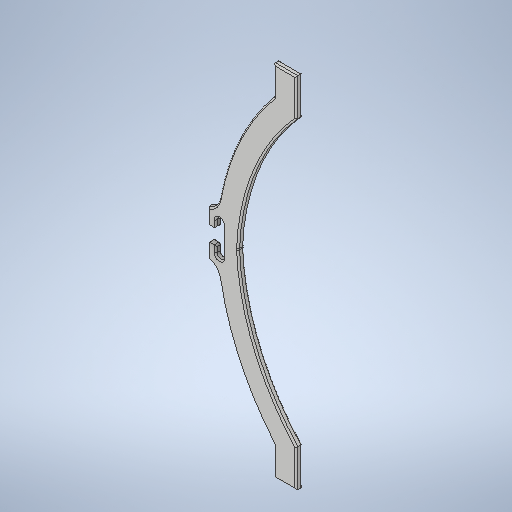
# Autodesk Inventor part: Baseplate_aussen_unten
Saved by Autodesk Inventor 2025 (Build 290162000, 162)
## iProperties
Created: 2020-01-15
Part Number: Baseplate_aussen_unten
Material: Generisch
Document SubType Name: Modeling
Designer: maxse
Density: 1 g/cm^3
Appearance: Vorgabe
Author: maxse
Autodesk Inventor part; units mm, degrees
ref_plane "YZ Plane" through (0, 0, 0) normal (1, 0, 0) x (0, 1, 0)
ref_plane "XZ Plane" through (0, 0, 0) normal (0, 1, 0) x (-1, 0, 0)
ref_plane "XY Plane" through (0, 0, 0) normal (0, 0, 1) x (1, 0, 0)
sketch "Skizze1" plane through (0, 0, 0) normal (0, 1, 0) x (-1, 0, 0)
  arc A0 (39, 0) -> (0, 95) centre (-110.879, -6.024) ccw
  line L0 (0, 95) -> (0, 120)
  line L1 (0, 120) -> (15, 120)
  line L2 (15, 120) -> (15, 100.6336)
  arc A1 (54, 0) -> (15, 100.6336) centre (-110.879, -6.024) ccw
  line L3 (39, 0) -> (54, 0)
  line L4 (0, 0) -> (39, 0)
  line L5 (59, 0) -> (59, 15)
  line L6 (59, 15) -> (52.765, 15)
  line L7 (59, 0) -> (54, 0)
  dimension "d0" = 25
  dimension "d2" = 15
  dimension "d4" = 54
  dimension "d5" = 0
  dimension "d6" = 120
  dimension "d7" = 150
  dimension "d9" = 5
  dimension "d10" = 15
  dimension "d11" = 15
  constraints: 16 end point, 6 point on circle, 3 perpendicular, 2 centre point, 2 horizontal, 2 vertical, 1 collinear, 1 concentric
  measures "d0" distance of L0.start L0.end
  measures "d2" distance of L0.end L1.end
  measures "d4" distance of L3.end L4.start
  measures "d5" distance from line of L4.start L0
  measures "d6" distance from line of L4.start L1
  measures "d7" radius of A0
  measures "d9" distance of L3.end L5.start
  measures "d10" distance of L3.end L3.start
  measures "d11" distance of L5.start L5.end
extrude "Extrusion1" add sketch "Skizze1" along normal blind 4
mirror "Spiegeln1" about plane through (-54, 0, 0) normal (0, 0, -1) of "Extrusion1"
sketch "Skizze2" plane through (0, 0, 0) normal (0, -1, 0) x (1, 0, 0)
  line L0 (-59, 15) -> (-59, -15) projected
  line L1 (-59, -5) -> (-54, -5)
  line L2 (-54, -5) -> (-54, -9.5)
  line L3 (-59, 5) -> (-54, 5)
  line L4 (-54, 5) -> (-54, 9.5)
  line L5 (-49, -9.5) -> (-49, 9.5)
  arc A0 (-49, 9.5) -> (-54, 9.5) centre (-51.5, 9.5) ccw
  arc A1 (-54, -9.5) -> (-49, -9.5) centre (-51.5, -9.5) ccw
  point P0 (0, 0)
  dimension "d15" = 10
  dimension "d16" = 5
  dimension "d17" = 10
  dimension "d18" = 5
  dimension "d19" = 5
  dimension "d20" = 24
  dimension "d21" = 4.5
  constraints: 10 end point, 4 point on circle, 4 tangent, 2 centre point, 2 horizontal, 2 point on line, 2 vertical, 1 perpendicular
  measures "d15" distance between parallel lines of L5 L0
  measures "d16" distance between parallel lines of L5 L2
  measures "d17" distance between parallel lines of L3 L1
  measures "d18" distance of L3.start L3.end
  measures "d19" distance from line of point (0, 0) L3
  measures "d21" distance from line of L1 A1.centre
extrude "Extrusion2" cut sketch "Skizze2" against normal blind 4
fillet "Rundung1" radius 10 3 edges at (-52.765, 2, -15) (-52.765, 2, 15) (-39, 2, 0)
fillet "Rundung2" radius 1 46 edges at (-7.5, 4, -120) (0, 4, -107.5) (-15, 4, -110.3168) (-7.5, 0, -120) (0, 0, -107.5) (-15, 0, -110.3168) (-54.0935, 4, -17.8718) (-38.4134, 4, -64.2123) (-54.0935, 0, -17.8718) (-38.4134, 0, -64.2123) (-38.9913, 4, 0) (-27.8012, 4, 51.1406) (-27.8012, 4, -51.1406) (-38.9913, 0, 0) (-27.8012, 0, 51.1406) (-27.8012, 0, -51.1406) (-54.0935, 4, 17.8718) (-38.4134, 4, 64.2123) (-54.0935, 0, 17.8718) (-38.4134, 0, 64.2123) (-59, 4, 10) (-59, 0, 10) (-59, 0, -10) (-59, 4, -10) (-59, 2, -5) (-59, 2, 5) (-54, 2, 5) (-54, 2, -5) (-56.5, 4, -5) (-56.5, 4, 5) (-51.5, 4, 12) (-54, 4, 7.25) (-51.5, 4, -12) (-54, 4, -7.25) (-49, 4, 0) (-51.5, 0, -12) (-54, 0, -7.25) (-51.5, 0, 12) (-54, 0, 7.25) (-49, 0, 0) (-15, 4, 110.3168) (-15, 0, 110.3168) (-7.5, 4, 120) (-7.5, 0, 120) (0, 0, 107.5) (0, 4, 107.5)
sketch "Skizze3" plane through (0, 4, 0) normal (0, 1, 0) x (1, 0, 0)
  arc A0 (0, 94.8126) -> (0, -95) centre (94.4443, -0.0937) ccw
  spline S0 degree 2 poles (-37.712, -45.9787) (-37.4072, -45.8685) (-36.7799, -45.8874) (-36.5192, -46.0129) knots 0 0 0 1 2 2 2
  spline S1 degree 2 poles (-36.5192, -46.0129) (-36.191, -46.17) (-35.705, -46.7397) (-35.5232, -47.2427) knots 0 0 0 1 2 2 2
  line L0 (-35.5232, -47.2427) -> (-35.3317, -47.7723)
  line L1 (-35.3317, -47.7723) -> (-33.5789, -47.1388)
  line L2 (-33.5789, -47.1388) -> (-33.353, -47.7637)
  line L3 (-33.353, -47.7637) -> (-38.0552, -49.4633)
  line L4 (-38.0552, -49.4633) -> (-38.4822, -48.282)
  spline S2 degree 2 poles (-38.4822, -48.282) (-38.6337, -47.8629) (-38.7087, -47.2265) (-38.6337, -46.9452) knots 0 0 0 1 2 2 2
  spline S3 degree 2 poles (-38.6337, -46.9452) (-38.5496, -46.6175) (-38.1045, -46.1206) (-37.712, -45.9787) knots 0 0 0 1 2 2 2
  spline S4 degree 2 poles (-37.4574, -46.6234) (-37.7013, -46.7116) (-37.9989, -47.0087) (-38.0513, -47.2215) knots 0 0 0 1 2 2 2
  spline S5 degree 2 poles (-38.0513, -47.2215) (-38.0966, -47.4059) (-38.0334, -47.8311) (-37.9273, -48.1246) knots 0 0 0 1 2 2 2
  line L5 (-37.9273, -48.1246) -> (-37.74, -48.6428)
  line L6 (-37.74, -48.6428) -> (-35.8652, -47.9652)
  line L7 (-35.8652, -47.9652) -> (-36.0195, -47.5384)
  spline S6 degree 2 poles (-36.0195, -47.5384) (-36.1572, -47.1573) (-36.4486, -46.7327) (-36.6637, -46.6381) knots 0 0 0 1 2 2 2
  spline S7 degree 2 poles (-36.6637, -46.6381) (-36.8557, -46.5481) (-37.2326, -46.5422) (-37.4574, -46.6234) knots 0 0 0 1 2 2 2
  spline S8 degree 2 poles (-35.6468, -42.3782) (-35.5687, -42.4335) (-35.2949, -42.616) (-35.199, -42.7123) knots 0 0 0 1 2 2 2
  spline S9 degree 2 poles (-35.199, -42.7123) (-35.0622, -42.842) (-34.8756, -43.1089) (-34.7865, -43.3781) knots 0 0 0 1 2 2 2
  spline S10 degree 2 poles (-34.7865, -43.3781) (-34.7139, -43.5974) (-34.7482, -44.0483) (-34.8485, -44.248) knots 0 0 0 1 2 2 2
  spline S11 degree 2 poles (-34.8485, -44.248) (-34.9476, -44.4387) (-35.3211, -44.7544) (-35.5596, -44.8334) knots 0 0 0 1 2 2 2
  spline S12 degree 2 poles (-35.5596, -44.8334) (-35.9288, -44.9556) (-36.5551, -44.8173) (-36.8172, -44.5284) knots 0 0 0 1 2 2 2
  spline S13 degree 2 poles (-36.8172, -44.5284) (-37.055, -44.2742) (-37.4288, -43.4932) (-37.6124, -43.0289) knots 0 0 0 1 2 2 2
  line L8 (-37.6124, -43.0289) -> (-37.7278, -43.0671)
  spline S14 degree 2 poles (-37.7278, -43.0671) (-37.9355, -43.1359) (-38.1512, -43.3482) (-38.1861, -43.4878) knots 0 0 0 1 2 2 2
  spline S15 degree 2 poles (-38.1861, -43.4878) (-38.2209, -43.6274) (-38.1576, -43.9734) (-38.099, -44.1504) knots 0 0 0 1 2 2 2
  spline S16 degree 2 poles (-38.099, -44.1504) (-38.0302, -44.3581) (-37.7212, -44.8789) (-37.509, -45.1203) knots 0 0 0 1 2 2 2
  line L9 (-37.509, -45.1203) -> (-37.4976, -45.1549)
  line L10 (-37.4976, -45.1549) -> (-38.1092, -45.3574)
  spline S17 degree 2 poles (-38.1092, -45.3574) (-38.2101, -45.2072) (-38.5305, -44.6261) (-38.6311, -44.3223) knots 0 0 0 1 2 2 2
  spline S18 degree 2 poles (-38.6311, -44.3223) (-38.7534, -43.953) (-38.8048, -43.4109) (-38.721, -43.1612) knots 0 0 0 1 2 2 2
  spline S19 degree 2 poles (-38.721, -43.1612) (-38.6398, -42.9166) (-38.238, -42.5702) (-37.9033, -42.4594) knots 0 0 0 1 2 2 2
  line L11 (-37.9033, -42.4594) -> (-35.4685, -41.6534)
  line L12 (-35.4685, -41.6534) -> (-35.2698, -42.2534)
  line L13 (-35.2698, -42.2534) -> (-35.6468, -42.3782)
  line L14 (-36.1468, -42.5438) -> (-37.1354, -42.871)
  spline S20 degree 2 poles (-37.1354, -42.871) (-37.0449, -43.0801) (-36.7642, -43.7085) (-36.6352, -43.892) knots 0 0 0 1 2 2 2
  spline S21 degree 2 poles (-36.6352, -43.892) (-36.4832, -44.1063) (-36.0761, -44.3172) (-35.8069, -44.2281) knots 0 0 0 1 2 2 2
  spline S22 degree 2 poles (-35.8069, -44.2281) (-35.4992, -44.1262) (-35.3022, -43.6769) (-35.4117, -43.3461) knots 0 0 0 1 2 2 2
  spline S23 degree 2 poles (-35.4117, -43.3461) (-35.5047, -43.0653) (-35.8998, -42.6839) (-36.1468, -42.5438) knots 0 0 0 1 2 2 2
  line L15 (-39.2549, -39.8049) -> (-39.2454, -39.8359)
  spline S24 degree 2 poles (-39.2454, -39.8359) (-39.2434, -39.9116) (-39.2049, -40.0651) (-39.1728, -40.1697) knots 0 0 0 1 2 2 2
  spline S25 degree 2 poles (-39.1728, -40.1697) (-39.098, -40.4137) (-38.7377, -40.8288) (-38.462, -40.9816) knots 0 0 0 1 2 2 2
  line L16 (-38.462, -40.9816) -> (-35.9168, -40.2016)
  line L17 (-35.9168, -40.2016) -> (-35.7316, -40.806)
  line L18 (-35.7316, -40.806) -> (-39.3189, -41.9054)
  line L19 (-39.3189, -41.9054) -> (-39.5042, -41.301)
  line L20 (-39.5042, -41.301) -> (-38.9695, -41.1372)
  spline S26 degree 2 poles (-38.9695, -41.1372) (-39.3649, -40.8981) (-39.7559, -40.4797) (-39.8271, -40.2473) knots 0 0 0 1 2 2 2
  spline S27 degree 2 poles (-39.8271, -40.2473) (-39.8556, -40.1543) (-39.8763, -40.0589) (-39.8825, -39.9973) knots 0 0 0 1 2 2 2
  line L21 (-39.8825, -39.9973) -> (-39.2549, -39.8049)
  line L22 (-36.6281, -37.8134) -> (-36.4518, -38.4205)
  line L23 (-36.4518, -38.4205) -> (-40.0551, -39.4665)
  line L24 (-40.0551, -39.4665) -> (-40.2313, -38.8594)
  line L25 (-40.2313, -38.8594) -> (-36.6281, -37.8134)
  line L26 (-40.843, -38.9906) -> (-40.6431, -39.6793)
  line L27 (-40.6431, -39.6793) -> (-41.2734, -39.8623)
  line L28 (-41.2734, -39.8623) -> (-41.4734, -39.1736)
  line L29 (-41.4734, -39.1736) -> (-40.843, -38.9906)
  spline S28 degree 2 poles (-37.0651, -35.9211) (-36.9663, -36.2847) (-36.9906, -36.9674) (-37.0437, -37.2044) knots 0 0 0 1 2 2 2
  line L30 (-37.0437, -37.2044) -> (-37.7279, -37.3905)
  line L31 (-37.7279, -37.3905) -> (-37.7364, -37.3592)
  spline S29 degree 2 poles (-37.7364, -37.3592) (-37.6951, -37.264) (-37.604, -37.0124) (-37.5697, -36.8142) knots 0 0 0 1 2 2 2
  spline S30 degree 2 poles (-37.5697, -36.8142) (-37.5369, -36.6415) (-37.5295, -36.2364) (-37.5837, -36.037) knots 0 0 0 1 2 2 2
  spline S31 degree 2 poles (-37.5837, -36.037) (-37.6231, -35.8923) (-37.7799, -35.578) (-37.8559, -35.5147) knots 0 0 0 1 2 2 2
  spline S32 degree 2 poles (-37.8559, -35.5147) (-37.961, -35.4215) (-38.1568, -35.3656) (-38.3288, -35.4124) knots 0 0 0 1 2 2 2
  spline S33 degree 2 poles (-38.3288, -35.4124) (-38.5439, -35.4709) (-38.7029, -35.766) (-38.6954, -36.0873) knots 0 0 0 1 2 2 2
  spline S34 degree 2 poles (-38.6954, -36.0873) (-38.6908, -36.212) (-38.667, -36.6087) (-38.6664, -36.7807) knots 0 0 0 1 2 2 2
  spline S35 degree 2 poles (-38.6664, -36.7807) (-38.6749, -37.2281) (-39.0733, -37.7395) (-39.4291, -37.8363) knots 0 0 0 1 2 2 2
  spline S36 degree 2 poles (-39.4291, -37.8363) (-39.9217, -37.9702) (-40.7365, -37.3982) (-40.9024, -36.7883) knots 0 0 0 1 2 2 2
  spline S37 degree 2 poles (-40.9024, -36.7883) (-40.9842, -36.4872) (-41.0015, -35.8369) (-40.9445, -35.5988) knots 0 0 0 1 2 2 2
  line L32 (-40.9445, -35.5988) -> (-40.2916, -35.4212)
  line L33 (-40.2916, -35.4212) -> (-40.283, -35.4525)
  spline S38 degree 2 poles (-40.283, -35.4525) (-40.4069, -35.7381) (-40.4667, -36.3675) (-40.387, -36.6607) knots 0 0 0 1 2 2 2
  spline S39 degree 2 poles (-40.387, -36.6607) (-40.3051, -36.9618) (-39.9383, -37.3071) (-39.6841, -37.238) knots 0 0 0 1 2 2 2
  spline S40 degree 2 poles (-39.6841, -37.238) (-39.4535, -37.1753) (-39.2976, -36.8683) (-39.3016, -36.5755) knots 0 0 0 1 2 2 2
  spline S41 degree 2 poles (-39.3016, -36.5755) (-39.3026, -36.433) (-39.3236, -36.0776) (-39.3306, -35.8821) knots 0 0 0 1 2 2 2
  spline S42 degree 2 poles (-39.3306, -35.8821) (-39.3374, -35.4557) (-38.9827, -34.9225) (-38.58, -34.813) knots 0 0 0 1 2 2 2
  spline S43 degree 2 poles (-38.58, -34.813) (-38.3454, -34.7492) (-37.881, -34.8203) (-37.6796, -34.9587) knots 0 0 0 1 2 2 2
  spline S44 degree 2 poles (-37.6796, -34.9587) (-37.4672, -35.1067) (-37.1661, -35.5497) (-37.0651, -35.9211) knots 0 0 0 1 2 2 2
  line L34 (-38.8586, -29.0048) -> (-38.2094, -31.8282)
  line L35 (-38.2094, -31.8282) -> (-43.0823, -32.9486)
  line L36 (-43.0823, -32.9486) -> (-43.2312, -32.301)
  line L37 (-43.2312, -32.301) -> (-38.9349, -31.3132)
  line L38 (-38.9349, -31.3132) -> (-39.4351, -29.1374)
  line L39 (-39.4351, -29.1374) -> (-38.8586, -29.0048)
  spline S45 degree 2 poles (-41.4057, -25.8908) (-40.4764, -25.7027) (-39.2828, -26.3912) (-39.1316, -27.1378) knots 0 0 0 1 2 2 2
  spline S46 degree 2 poles (-39.1316, -27.1378) (-38.9765, -27.9042) (-39.8432, -28.9934) (-40.7407, -29.1751) knots 0 0 0 1 2 2 2
  spline S47 degree 2 poles (-40.7407, -29.1751) (-41.662, -29.3616) (-42.866, -28.6628) (-43.0156, -27.9242) knots 0 0 0 1 2 2 2
  spline S48 degree 2 poles (-43.0156, -27.9242) (-43.1667, -27.1776) (-42.331, -26.0782) (-41.4057, -25.8908) knots 0 0 0 1 2 2 2
  spline S49 degree 2 poles (-41.2762, -26.5302) (-41.9911, -26.675) (-42.5807, -27.3359) (-42.4834, -27.8164) knots 0 0 0 1 2 2 2
  spline S50 degree 2 poles (-42.4834, -27.8164) (-42.3861, -28.297) (-41.585, -28.6805) (-40.8702, -28.5357) knots 0 0 0 1 2 2 2
  spline S51 degree 2 poles (-40.8702, -28.5357) (-40.1752, -28.395) (-39.5665, -27.7261) (-39.6638, -27.2455) knots 0 0 0 1 2 2 2
  spline S52 degree 2 poles (-39.6638, -27.2455) (-39.7603, -26.769) (-40.5693, -26.3871) (-41.2762, -26.5302) knots 0 0 0 1 2 2 2
  line L40 (-40.1779, -22.0386) -> (-40.0696, -22.6614)
  line L41 (-40.0696, -22.6614) -> (-40.4449, -22.7266)
  spline S53 degree 2 poles (-40.4449, -22.7266) (-40.3001, -22.8495) (-40.1037, -23.0333) (-40.0108, -23.1652) knots 0 0 0 1 2 2 2
  spline S54 degree 2 poles (-40.0108, -23.1652) (-39.924, -23.2859) (-39.8069, -23.5575) (-39.7743, -23.7451) knots 0 0 0 1 2 2 2
  spline S55 degree 2 poles (-39.7743, -23.7451) (-39.7215, -24.0485) (-39.8841, -24.6032) (-40.0964, -24.8252) knots 0 0 0 1 2 2 2
  spline S56 degree 2 poles (-40.0964, -24.8252) (-40.3087, -25.0472) (-40.9925, -25.3717) (-41.4596, -25.4529) knots 0 0 0 1 2 2 2
  spline S57 degree 2 poles (-41.4596, -25.4529) (-41.9466, -25.5376) (-42.7009, -25.4097) (-43.0066, -25.2366) knots 0 0 0 1 2 2 2
  spline S58 degree 2 poles (-43.0066, -25.2366) (-43.2815, -25.0747) (-43.6562, -24.5517) (-43.711, -24.2364) knots 0 0 0 1 2 2 2
  spline S59 degree 2 poles (-43.711, -24.2364) (-43.7589, -23.9609) (-43.7067, -23.5282) (-43.6185, -23.2785) knots 0 0 0 1 2 2 2
  line L42 (-43.6185, -23.2785) -> (-45.2153, -23.5561)
  line L43 (-45.2153, -23.5561) -> (-45.3236, -22.9334)
  line L44 (-45.3236, -22.9334) -> (-40.1779, -22.0386)
  line L45 (-40.9678, -22.8176) -> (-43.1035, -23.1889)
  spline S60 degree 2 poles (-43.1035, -23.1889) (-43.175, -23.4399) (-43.195, -23.8217) (-43.1582, -24.0333) knots 0 0 0 1 2 2 2
  spline S61 degree 2 poles (-43.1582, -24.0333) (-43.0749, -24.5123) (-42.262, -24.9303) (-41.5833, -24.8123) knots 0 0 0 1 2 2 2
  spline S62 degree 2 poles (-41.5833, -24.8123) (-40.9287, -24.6985) (-40.3102, -24.1632) (-40.3901, -23.7041) knots 0 0 0 1 2 2 2
  spline S63 degree 2 poles (-40.3901, -23.7041) (-40.4324, -23.4606) (-40.742, -23.0045) (-40.9678, -22.8176) knots 0 0 0 1 2 2 2
  line L46 (-43.6537, -19.6231) -> (-43.6489, -19.6552)
  spline S64 degree 2 poles (-43.6489, -19.6552) (-43.6581, -19.7303) (-43.6426, -19.8878) (-43.6264, -19.996) knots 0 0 0 1 2 2 2
  spline S65 degree 2 poles (-43.6264, -19.996) (-43.5885, -20.2484) (-43.2934, -20.7122) (-43.0433, -20.904) knots 0 0 0 1 2 2 2
  line L47 (-43.0433, -20.904) -> (-40.4108, -20.5085)
  line L48 (-40.4108, -20.5085) -> (-40.3169, -21.1336)
  line L49 (-40.3169, -21.1336) -> (-44.0273, -21.6911)
  line L50 (-44.0273, -21.6911) -> (-44.1212, -21.066)
  line L51 (-44.1212, -21.066) -> (-43.5682, -20.9829)
  spline S66 degree 2 poles (-43.5682, -20.9829) (-43.9239, -20.6881) (-44.2488, -20.2165) (-44.285, -19.9761) knots 0 0 0 1 2 2 2
  spline S67 degree 2 poles (-44.285, -19.9761) (-44.2994, -19.88) (-44.3058, -19.7826) (-44.3028, -19.7207) knots 0 0 0 1 2 2 2
  line L52 (-44.3028, -19.7207) -> (-43.6537, -19.6231)
  spline S68 degree 2 poles (-42.9318, -15.8585) (-41.9912, -15.739) (-40.8513, -16.5131) (-40.7553, -17.2688) knots 0 0 0 1 2 2 2
  spline S69 degree 2 poles (-40.7553, -17.2688) (-40.6567, -18.0446) (-41.601, -19.0672) (-42.5094, -19.1826) knots 0 0 0 1 2 2 2
  spline S70 degree 2 poles (-42.5094, -19.1826) (-43.442, -19.3011) (-44.5914, -18.5159) (-44.6864, -17.7683) knots 0 0 0 1 2 2 2
  spline S71 degree 2 poles (-44.6864, -17.7683) (-44.7824, -17.0126) (-43.8683, -15.9775) (-42.9318, -15.8585) knots 0 0 0 1 2 2 2
  spline S72 degree 2 poles (-42.8496, -16.5056) (-43.5731, -16.5975) (-44.2096, -17.2135) (-44.1478, -17.6998) knots 0 0 0 1 2 2 2
  spline S73 degree 2 poles (-44.1478, -17.6998) (-44.086, -18.1862) (-43.3152, -18.6274) (-42.5917, -18.5355) knots 0 0 0 1 2 2 2
  spline S74 degree 2 poles (-42.5917, -18.5355) (-41.8882, -18.4461) (-41.2321, -17.8236) (-41.2939, -17.3373) knots 0 0 0 1 2 2 2
  spline S75 degree 2 poles (-41.2939, -17.3373) (-41.3552, -16.8549) (-42.1341, -16.4147) (-42.8496, -16.5056) knots 0 0 0 1 2 2 2
  line L53 (-41.4306, -12.0462) -> (-41.3684, -12.6752)
  line L54 (-41.3684, -12.6752) -> (-43.4973, -12.8859)
  spline S76 degree 2 poles (-43.4973, -12.8859) (-43.7554, -12.9114) (-44.1942, -13.0037) (-44.32, -13.0894) knots 0 0 0 1 2 2 2
  spline S77 degree 2 poles (-44.32, -13.0894) (-44.4536, -13.18) (-44.5635, -13.4678) (-44.5404, -13.7016) knots 0 0 0 1 2 2 2
  spline S78 degree 2 poles (-44.5404, -13.7016) (-44.5173, -13.9355) (-44.2182, -14.4067) (-43.993, -14.6247) knots 0 0 0 1 2 2 2
  line L55 (-43.993, -14.6247) -> (-41.2028, -14.3485)
  line L56 (-41.2028, -14.3485) -> (-41.1405, -14.9776)
  line L57 (-41.1405, -14.9776) -> (-44.8743, -15.3471)
  line L58 (-44.8743, -15.3471) -> (-44.9365, -14.718)
  line L59 (-44.9365, -14.718) -> (-44.5212, -14.6769)
  spline S79 degree 2 poles (-44.5212, -14.6769) (-44.8032, -14.4198) (-45.1232, -13.9018) (-45.1535, -13.5954) knots 0 0 0 1 2 2 2
  spline S80 degree 2 poles (-45.1535, -13.5954) (-45.2078, -13.047) (-44.5434, -12.3542) (-43.8539, -12.286) knots 0 0 0 1 2 2 2
  line L60 (-43.8539, -12.286) -> (-41.4306, -12.0462)
  spline S81 degree 2 poles (-41.6553, -7.2225) (-41.6322, -7.6636) (-41.8285, -8.3312) (-42.0471, -8.5739) knots 0 0 0 1 2 2 2
  spline S82 degree 2 poles (-42.0471, -8.5739) (-42.2923, -8.8505) (-43.0094, -9.103) (-43.5435, -9.131) knots 0 0 0 1 2 2 2
  line L61 (-43.5435, -9.131) -> (-46.6591, -9.2942)
  line L62 (-46.6591, -9.2942) -> (-46.6939, -8.6306)
  line L63 (-46.6939, -8.6306) -> (-43.5782, -8.4674)
  spline S83 degree 2 poles (-43.5782, -8.4674) (-43.2302, -8.4492) (-42.7655, -8.3356) (-42.5819, -8.2002) knots 0 0 0 1 2 2 2
  spline S84 degree 2 poles (-42.5819, -8.2002) (-42.3866, -8.0561) (-42.2044, -7.584) (-42.2218, -7.2522) knots 0 0 0 1 2 2 2
  spline S85 degree 2 poles (-42.2218, -7.2522) (-42.2381, -6.9406) (-42.4699, -6.4659) (-42.6792, -6.3429) knots 0 0 0 1 2 2 2
  spline S86 degree 2 poles (-42.6792, -6.3429) (-42.8759, -6.2275) (-43.3459, -6.1628) (-43.6818, -6.1804) knots 0 0 0 1 2 2 2
  line L64 (-43.6818, -6.1804) -> (-46.8136, -6.3444)
  line L65 (-46.8136, -6.3444) -> (-46.8484, -5.6808)
  line L66 (-46.8484, -5.6808) -> (-43.7327, -5.5177)
  spline S87 degree 2 poles (-43.7327, -5.5177) (-43.2107, -5.4903) (-42.4552, -5.6617) (-42.1863, -5.9155) knots 0 0 0 1 2 2 2
  spline S88 degree 2 poles (-42.1863, -5.9155) (-41.9391, -6.1419) (-41.6794, -6.7613) (-41.6553, -7.2225) knots 0 0 0 1 2 2 2
  line L67 (-41.9473, -1.5713) -> (-41.9336, -2.2032)
  line L68 (-41.9336, -2.2032) -> (-44.0725, -2.2497)
  spline S89 degree 2 poles (-44.0725, -2.2497) (-44.3317, -2.2554) (-44.7763, -2.3137) (-44.9083, -2.3895) knots 0 0 0 1 2 2 2
  spline S90 degree 2 poles (-44.9083, -2.3895) (-45.0485, -2.4695) (-45.1802, -2.748) (-45.1751, -2.9829) knots 0 0 0 1 2 2 2
  spline S91 degree 2 poles (-45.1751, -2.9829) (-45.17, -3.2179) (-44.908, -3.7107) (-44.7003, -3.9453) knots 0 0 0 1 2 2 2
  line L69 (-44.7003, -3.9453) -> (-41.897, -3.8844)
  line L70 (-41.897, -3.8844) -> (-41.8833, -4.5163)
  line L71 (-41.8833, -4.5163) -> (-45.6344, -4.5979)
  line L72 (-45.6344, -4.5979) -> (-45.6482, -3.9659)
  line L73 (-45.6482, -3.9659) -> (-45.2309, -3.9568)
  spline S92 degree 2 poles (-45.2309, -3.9568) (-45.4923, -3.6788) (-45.7715, -3.1378) (-45.7782, -2.8299) knots 0 0 0 1 2 2 2
  spline S93 degree 2 poles (-45.7782, -2.8299) (-45.7902, -2.279) (-45.0746, -1.6393) (-44.3819, -1.6242) knots 0 0 0 1 2 2 2
  line L74 (-44.3819, -1.6242) -> (-41.9473, -1.5713)
  line L75 (-41.9476, -0.0397) -> (-41.9463, -0.6718)
  line L76 (-41.9463, -0.6718) -> (-45.6984, -0.679)
  line L77 (-45.6984, -0.679) -> (-45.6996, -0.0469)
  line L78 (-45.6996, -0.0469) -> (-41.9476, -0.0397)
  line L79 (-46.3237, -0.0035) -> (-46.3223, -0.7207)
  line L80 (-46.3223, -0.7207) -> (-46.9787, -0.722)
  line L81 (-46.9787, -0.722) -> (-46.9801, -0.0048)
  line L82 (-46.9801, -0.0048) -> (-46.3237, -0.0035)
  line L83 (-45.6527, 3.8949) -> (-41.9243, 2.4195)
  line L84 (-41.9243, 2.4195) -> (-41.9336, 1.8524)
  line L85 (-41.9336, 1.8524) -> (-45.7081, 0.5121)
  line L86 (-45.7081, 0.5121) -> (-45.6969, 1.1968)
  line L87 (-45.6969, 1.1968) -> (-42.7915, 2.1744)
  line L88 (-42.7915, 2.1744) -> (-45.6634, 3.2386)
  line L89 (-45.6634, 3.2386) -> (-45.6527, 3.8949)
  spline S94 degree 2 poles (-41.729, 5.935) (-41.767, 5.0363) (-42.8167, 4.0911) (-43.7478, 4.1304) knots 0 0 0 1 2 2 2
  spline S95 degree 2 poles (-43.7478, 4.1304) (-44.6627, 4.169) (-45.7071, 5.1743) (-45.6745, 5.9475) knots 0 0 0 1 2 2 2
  spline S96 degree 2 poles (-45.6745, 5.9475) (-45.6598, 6.2957) (-45.4346, 6.8255) (-45.2117, 7.0148) knots 0 0 0 1 2 2 2
  spline S97 degree 2 poles (-45.2117, 7.0148) (-44.9886, 7.2082) (-44.3601, 7.3966) (-43.9108, 7.3776) knots 0 0 0 1 2 2 2
  line L90 (-43.9108, 7.3776) -> (-43.5667, 7.3631)
  line L91 (-43.5667, 7.3631) -> (-43.6763, 4.7682)
  spline S98 degree 2 poles (-43.6763, 4.7682) (-43.0245, 4.7406) (-42.3045, 5.3672) (-42.2799, 5.9502) knots 0 0 0 1 2 2 2
  spline S99 degree 2 poles (-42.2799, 5.9502) (-42.2712, 6.1566) (-42.3474, 6.5613) (-42.4134, 6.7263) knots 0 0 0 1 2 2 2
  spline S100 degree 2 poles (-42.4134, 6.7263) (-42.4872, 6.8998) (-42.619, 7.1406) (-42.6805, 7.2202) knots 0 0 0 1 2 2 2
  line L92 (-42.6805, 7.2202) -> (-42.679, 7.2566)
  line L93 (-42.679, 7.2566) -> (-41.9908, 7.2276)
  spline S101 degree 2 poles (-41.9908, 7.2276) (-41.9508, 7.1164) (-41.8353, 6.779) (-41.8043, 6.6479) knots 0 0 0 1 2 2 2
  spline S102 degree 2 poles (-41.8043, 6.6479) (-41.7594, 6.4635) (-41.7194, 6.1617) (-41.729, 5.935) knots 0 0 0 1 2 2 2
  spline S103 degree 2 poles (-44.0744, 6.7681) (-44.3298, 6.7708) (-44.7067, 6.6812) (-44.8364, 6.5853) knots 0 0 0 1 2 2 2
  spline S104 degree 2 poles (-44.8364, 6.5853) (-44.9827, 6.482) (-45.1471, 6.1442) (-45.1578, 5.8892) knots 0 0 0 1 2 2 2
  spline S105 degree 2 poles (-45.1578, 5.8892) (-45.1684, 5.6382) (-45.0335, 5.2797) (-44.8939, 5.1278) knots 0 0 0 1 2 2 2
  spline S106 degree 2 poles (-44.8939, 5.1278) (-44.7501, 4.9798) (-44.396, 4.8188) (-44.158, 4.7885) knots 0 0 0 1 2 2 2
  line L94 (-44.158, 4.7885) -> (-44.0744, 6.7681)
  line L95 (-44.6541, 10.1091) -> (-44.6562, 10.0768)
  spline S107 degree 2 poles (-44.6562, 10.0768) (-44.6811, 10.0053) (-44.6994, 9.8481) (-44.7065, 9.739) knots 0 0 0 1 2 2 2
  spline S108 degree 2 poles (-44.7065, 9.739) (-44.7229, 9.4842) (-44.533, 8.9685) (-44.3293, 8.7279) knots 0 0 0 1 2 2 2
  line L96 (-44.3293, 8.7279) -> (-41.6727, 8.5562)
  line L97 (-41.6727, 8.5562) -> (-41.7135, 7.9254)
  line L98 (-41.7135, 7.9254) -> (-45.4577, 8.1675)
  line L99 (-45.4577, 8.1675) -> (-45.4169, 8.7982)
  line L100 (-45.4169, 8.7982) -> (-44.8589, 8.7622)
  spline S109 degree 2 poles (-44.8589, 8.7622) (-45.144, 9.1257) (-45.3615, 9.6554) (-45.3458, 9.898) knots 0 0 0 1 2 2 2
  spline S110 degree 2 poles (-45.3458, 9.898) (-45.3396, 9.9951) (-45.3252, 10.0916) (-45.3091, 10.1515) knots 0 0 0 1 2 2 2
  line L101 (-45.3091, 10.1515) -> (-44.6541, 10.1091)
  spline S111 degree 2 poles (-41.3725, 11.4012) (-41.4045, 11.0258) (-41.6616, 10.393) (-41.7929, 10.1886) knots 0 0 0 1 2 2 2
  line L102 (-41.7929, 10.1886) -> (-42.4994, 10.2487)
  line L103 (-42.4994, 10.2487) -> (-42.4967, 10.281)
  spline S112 degree 2 poles (-42.4967, 10.281) (-42.4252, 10.3563) (-42.2532, 10.5612) (-42.153, 10.7357) knots 0 0 0 1 2 2 2
  spline S113 degree 2 poles (-42.153, 10.7357) (-42.0629, 10.8866) (-41.9169, 11.2646) (-41.8993, 11.4705) knots 0 0 0 1 2 2 2
  spline S114 degree 2 poles (-41.8993, 11.4705) (-41.8866, 11.6199) (-41.926, 11.9689) (-41.9757, 12.0544) knots 0 0 0 1 2 2 2
  spline S115 degree 2 poles (-41.9757, 12.0544) (-42.0424, 12.178) (-42.2071, 12.2978) (-42.3848, 12.3129) knots 0 0 0 1 2 2 2
  spline S116 degree 2 poles (-42.3848, 12.3129) (-42.6068, 12.3318) (-42.8575, 12.1091) (-42.9607, 11.8048) knots 0 0 0 1 2 2 2
  spline S117 degree 2 poles (-42.9607, 11.8048) (-42.9993, 11.6861) (-43.113, 11.3054) (-43.1715, 11.1436) knots 0 0 0 1 2 2 2
  spline S118 degree 2 poles (-43.1715, 11.1436) (-43.3331, 10.7263) (-43.8828, 10.3827) (-44.2502, 10.414) knots 0 0 0 1 2 2 2
  spline S119 degree 2 poles (-44.2502, 10.414) (-44.7589, 10.4573) (-45.3278, 11.2743) (-45.2742, 11.9041) knots 0 0 0 1 2 2 2
  spline S120 degree 2 poles (-45.2742, 11.9041) (-45.2478, 12.2149) (-45.0408, 12.8317) (-44.9055, 13.0357) knots 0 0 0 1 2 2 2
  line L104 (-44.9055, 13.0357) -> (-44.2312, 12.9783)
  line L105 (-44.2312, 12.9783) -> (-44.234, 12.946)
  spline S121 degree 2 poles (-44.234, 12.946) (-44.4484, 12.7203) (-44.7206, 12.1497) (-44.7464, 11.847) knots 0 0 0 1 2 2 2
  spline S122 degree 2 poles (-44.7464, 11.847) (-44.7728, 11.5361) (-44.5468, 11.0858) (-44.2844, 11.0635) knots 0 0 0 1 2 2 2
  spline S123 degree 2 poles (-44.2844, 11.0635) (-44.0462, 11.0432) (-43.7944, 11.278) (-43.6977, 11.5544) knots 0 0 0 1 2 2 2
  spline S124 degree 2 poles (-43.6977, 11.5544) (-43.6497, 11.6886) (-43.5475, 12.0296) (-43.4869, 12.2156) knots 0 0 0 1 2 2 2
  spline S125 degree 2 poles (-43.4869, 12.2156) (-43.3469, 12.6184) (-42.8307, 12.9974) (-42.4149, 12.962) knots 0 0 0 1 2 2 2
  spline S126 degree 2 poles (-42.4149, 12.962) (-42.1727, 12.9414) (-41.7609, 12.7152) (-41.6192, 12.5161) knots 0 0 0 1 2 2 2
  spline S127 degree 2 poles (-41.6192, 12.5161) (-41.4705, 12.3042) (-41.3399, 11.7848) (-41.3725, 11.4012) knots 0 0 0 1 2 2 2
  line L106 (-41.2075, 14.0953) -> (-41.2718, 13.4665)
  line L107 (-41.2718, 13.4665) -> (-45.0044, 13.8481)
  line L108 (-45.0044, 13.8481) -> (-44.9401, 14.4769)
  line L109 (-44.9401, 14.4769) -> (-41.2075, 14.0953)
  line L110 (-45.5563, 14.5848) -> (-45.6293, 13.8713)
  line L111 (-45.6293, 13.8713) -> (-46.2823, 13.9381)
  line L112 (-46.2823, 13.9381) -> (-46.2093, 14.6515)
  line L113 (-46.2093, 14.6515) -> (-45.5563, 14.5848)
  spline S128 degree 2 poles (-40.9054, 16.1363) (-40.965, 15.6252) (-41.6157, 15.1178) (-42.2475, 15.1914) knots 0 0 0 1 2 2 2
  line L114 (-42.2475, 15.1914) -> (-44.3121, 15.4322)
  line L115 (-44.3121, 15.4322) -> (-44.3614, 15.0097)
  line L116 (-44.3614, 15.0097) -> (-44.8806, 15.0702)
  line L117 (-44.8806, 15.0702) -> (-44.8313, 15.4928)
  line L118 (-44.8313, 15.4928) -> (-45.9019, 15.6176)
  line L119 (-45.9019, 15.6176) -> (-45.8286, 16.2455)
  line L120 (-45.8286, 16.2455) -> (-44.7581, 16.1206)
  line L121 (-44.7581, 16.1206) -> (-44.6234, 17.2757)
  line L122 (-44.6234, 17.2757) -> (-44.1042, 17.2151)
  line L123 (-44.1042, 17.2151) -> (-44.2389, 16.0601)
  line L124 (-44.2389, 16.0601) -> (-42.4641, 15.8531)
  spline S129 degree 2 poles (-42.4641, 15.8531) (-42.1824, 15.8202) (-41.8701, 15.8042) (-41.7293, 15.8571) knots 0 0 0 1 2 2 2
  spline S130 degree 2 poles (-41.7293, 15.8571) (-41.606, 15.8999) (-41.4598, 16.1398) (-41.4344, 16.3571) knots 0 0 0 1 2 2 2
  spline S131 degree 2 poles (-41.4344, 16.3571) (-41.4166, 16.5101) (-41.4758, 16.8066) (-41.4965, 16.8743) knots 0 0 0 1 2 2 2
  line L125 (-41.4965, 16.8743) -> (-41.4923, 16.9105)
  line L126 (-41.4923, 16.9105) -> (-40.9288, 16.8448)
  spline S132 degree 2 poles (-40.9288, 16.8448) (-40.9012, 16.6621) (-40.8871, 16.2933) (-40.9054, 16.1363) knots 0 0 0 1 2 2 2
  line L127 (-44.1532, 20.7342) -> (-39.3434, 18.0337)
  line L128 (-39.3434, 18.0337) -> (-39.4359, 17.3634)
  line L129 (-39.4359, 17.3634) -> (-40.8933, 18.2435)
  line L130 (-40.8933, 18.2435) -> (-44.6156, 17.3826)
  line L131 (-44.6156, 17.3826) -> (-44.5225, 18.057)
  line L132 (-44.5225, 18.057) -> (-41.629, 18.6926)
  line L133 (-41.629, 18.6926) -> (-44.2429, 20.084)
  line L134 (-44.2429, 20.084) -> (-44.1532, 20.7342)
  spline S133 degree 2 poles (-39.6726, 24.2169) (-39.7695, 23.6826) (-40.1287, 22.9736) (-40.3481, 22.6716) knots 0 0 0 1 2 2 2
  line L135 (-40.3481, 22.6716) -> (-41.1694, 22.8206)
  line L136 (-41.1694, 22.8206) -> (-41.1608, 22.8684)
  spline S134 degree 2 poles (-41.1608, 22.8684) (-40.7992, 23.1364) (-40.3161, 23.893) (-40.2474, 24.2717) knots 0 0 0 1 2 2 2
  spline S135 degree 2 poles (-40.2474, 24.2717) (-40.149, 24.8139) (-40.499, 25.4498) (-40.8698, 25.5171) knots 0 0 0 1 2 2 2
  spline S136 degree 2 poles (-40.8698, 25.5171) (-41.1648, 25.5706) (-41.5844, 25.346) (-41.7332, 25.0477) knots 0 0 0 1 2 2 2
  spline S137 degree 2 poles (-41.7332, 25.0477) (-41.8382, 24.832) (-41.9946, 24.4692) (-42.1177, 24.1992) knots 0 0 0 1 2 2 2
  spline S138 degree 2 poles (-42.1177, 24.1992) (-42.2318, 23.9563) (-42.5081, 23.5905) (-42.6998, 23.4647) knots 0 0 0 1 2 2 2
  spline S139 degree 2 poles (-42.6998, 23.4647) (-42.8907, 23.3428) (-43.3597, 23.2549) (-43.6467, 23.307) knots 0 0 0 1 2 2 2
  spline S140 degree 2 poles (-43.6467, 23.307) (-44.2447, 23.4154) (-44.8849, 24.4951) (-44.754, 25.2167) knots 0 0 0 1 2 2 2
  spline S141 degree 2 poles (-44.754, 25.2167) (-44.6788, 25.6314) (-44.3823, 26.3353) (-44.1697, 26.6221) knots 0 0 0 1 2 2 2
  line L137 (-44.1697, 26.6221) -> (-43.3882, 26.4803)
  line L138 (-43.3882, 26.4803) -> (-43.3969, 26.4325)
  spline S142 degree 2 poles (-43.3969, 26.4325) (-43.6549, 26.2363) (-44.1069, 25.5606) (-44.1799, 25.1579) knots 0 0 0 1 2 2 2
  spline S143 degree 2 poles (-44.1799, 25.1579) (-44.2623, 24.7034) (-43.9377, 24.0639) (-43.5908, 24.001) knots 0 0 0 1 2 2 2
  spline S144 degree 2 poles (-43.5908, 24.001) (-43.2799, 23.9446) (-42.8491, 24.2083) (-42.7089, 24.504) knots 0 0 0 1 2 2 2
  spline S145 degree 2 poles (-42.7089, 24.504) (-42.6155, 24.7012) (-42.3628, 25.2772) (-42.2669, 25.4657) knots 0 0 0 1 2 2 2
  spline S146 degree 2 poles (-42.2669, 25.4657) (-42.0195, 25.9438) (-41.3083, 26.3008) (-40.8498, 26.2176) knots 0 0 0 1 2 2 2
  spline S147 degree 2 poles (-40.8498, 26.2176) (-40.5588, 26.1648) (-40.0433, 25.8284) (-39.8862, 25.5816) knots 0 0 0 1 2 2 2
  spline S148 degree 2 poles (-39.8862, 25.5816) (-39.7136, 25.3074) (-39.5908, 24.6674) (-39.6726, 24.2169) knots 0 0 0 1 2 2 2
  spline S149 degree 2 poles (-39.2802, 28.7061) (-39.2405, 28.6191) (-39.0954, 28.3237) (-39.0609, 28.1923) knots 0 0 0 1 2 2 2
  spline S150 degree 2 poles (-39.0609, 28.1923) (-39.0077, 28.0114) (-38.9806, 27.6869) (-39.0388, 27.4093) knots 0 0 0 1 2 2 2
  spline S151 degree 2 poles (-39.0388, 27.4093) (-39.0862, 27.1833) (-39.3423, 26.8106) (-39.5294, 26.6884) knots 0 0 0 1 2 2 2
  spline S152 degree 2 poles (-39.5294, 26.6884) (-39.7109, 26.5732) (-40.1924, 26.4879) (-40.4383, 26.5395) knots 0 0 0 1 2 2 2
  spline S153 degree 2 poles (-40.4383, 26.5395) (-40.819, 26.6193) (-41.291, 27.0536) (-41.3725, 27.435) knots 0 0 0 1 2 2 2
  spline S154 degree 2 poles (-41.3725, 27.435) (-41.4504, 27.7743) (-41.3812, 28.6374) (-41.3066, 29.131) knots 0 0 0 1 2 2 2
  line L139 (-41.3066, 29.131) -> (-41.4256, 29.156)
  spline S155 degree 2 poles (-41.4256, 29.156) (-41.6398, 29.2009) (-41.9329, 29.1257) (-42.0332, 29.0225) knots 0 0 0 1 2 2 2
  spline S156 degree 2 poles (-42.0332, 29.0225) (-42.1335, 28.9194) (-42.2526, 28.5883) (-42.2908, 28.4059) knots 0 0 0 1 2 2 2
  spline S157 degree 2 poles (-42.2908, 28.4059) (-42.3357, 28.1917) (-42.3302, 27.5861) (-42.268, 27.2709) knots 0 0 0 1 2 2 2
  line L140 (-42.268, 27.2709) -> (-42.2755, 27.2352)
  line L141 (-42.2755, 27.2352) -> (-42.906, 27.3674)
  spline S158 degree 2 poles (-42.906, 27.3674) (-42.9178, 27.5479) (-42.9029, 28.2113) (-42.8372, 28.5246) knots 0 0 0 1 2 2 2
  spline S159 degree 2 poles (-42.8372, 28.5246) (-42.7574, 28.9053) (-42.5295, 29.3998) (-42.3316, 29.5736) knots 0 0 0 1 2 2 2
  spline S160 degree 2 poles (-42.3316, 29.5736) (-42.1385, 29.7443) (-41.6171, 29.8419) (-41.2721, 29.7696) knots 0 0 0 1 2 2 2
  line L142 (-41.2721, 29.7696) -> (-38.7619, 29.2432)
  line L143 (-38.7619, 29.2432) -> (-38.8916, 28.6246)
  line L144 (-38.8916, 28.6246) -> (-39.2802, 28.7061)
  line L145 (-39.7957, 28.8142) -> (-40.8149, 29.0279)
  spline S161 degree 2 poles (-40.8149, 29.0279) (-40.8416, 28.8017) (-40.9148, 28.1173) (-40.8954, 27.8939) knots 0 0 0 1 2 2 2
  spline S162 degree 2 poles (-40.8954, 27.8939) (-40.8716, 27.6322) (-40.6257, 27.2453) (-40.3481, 27.1871) knots 0 0 0 1 2 2 2
  spline S163 degree 2 poles (-40.3481, 27.1871) (-40.0308, 27.1206) (-39.6348, 27.4101) (-39.5632, 27.7511) knots 0 0 0 1 2 2 2
  spline S164 degree 2 poles (-39.5632, 27.7511) (-39.5025, 28.0406) (-39.6526, 28.5689) (-39.7957, 28.8142) knots 0 0 0 1 2 2 2
  line L146 (-38.4176, 30.7356) -> (-38.5591, 30.1196)
  line L147 (-38.5591, 30.1196) -> (-43.6495, 31.2883)
  line L148 (-43.6495, 31.2883) -> (-43.508, 31.9044)
  line L149 (-43.508, 31.9044) -> (-38.4176, 30.7356)
  line L150 (-37.6166, 34.031) -> (-38.2787, 31.3564)
  line L151 (-38.2787, 31.3564) -> (-38.7349, 31.4694)
  line L152 (-38.7349, 31.4694) -> (-40.9461, 34.037)
  line L153 (-40.9461, 34.037) -> (-41.3979, 32.212)
  line L154 (-41.3979, 32.212) -> (-41.9013, 32.3366)
  line L155 (-41.9013, 32.3366) -> (-41.2675, 34.8971)
  line L156 (-41.2675, 34.8971) -> (-40.8309, 34.7891)
  line L157 (-40.8309, 34.7891) -> (-38.6138, 32.2116)
  line L158 (-38.6138, 32.2116) -> (-38.1319, 34.1585)
  line L159 (-38.1319, 34.1585) -> (-37.6166, 34.031)
  spline S165 degree 2 poles (-38.5037, 38.1482) (-37.6167, 37.9048) (-36.7702, 36.7482) (-36.9482, 36.0995) knots 0 0 0 1 2 2 2
  spline S166 degree 2 poles (-36.9482, 36.0995) (-37.0286, 35.8065) (-37.2879, 35.428) (-37.4687, 35.2592) knots 0 0 0 1 2 2 2
  line L160 (-37.4687, 35.2592) -> (-37.3114, 35.174)
  line L161 (-37.3114, 35.174) -> (-37.4679, 34.6035)
  line L162 (-37.4679, 34.6035) -> (-42.5046, 35.9854)
  line L163 (-42.5046, 35.9854) -> (-42.3374, 36.595)
  line L164 (-42.3374, 36.595) -> (-40.5399, 36.1018)
  spline S167 degree 2 poles (-40.5399, 36.1018) (-40.6838, 36.3892) (-40.8104, 36.9996) (-40.7171, 37.3395) knots 0 0 0 1 2 2 2
  spline S168 degree 2 poles (-40.7171, 37.3395) (-40.5488, 37.953) (-39.3751, 38.3872) (-38.5037, 38.1482) knots 0 0 0 1 2 2 2
  spline S169 degree 2 poles (-38.6294, 37.5062) (-39.2781, 37.6842) (-40.0584, 37.4739) (-40.1785, 37.0363) knots 0 0 0 1 2 2 2
  spline S170 degree 2 poles (-40.1785, 37.0363) (-40.2461, 36.7901) (-40.151, 36.2178) (-40.0281, 35.9614) knots 0 0 0 1 2 2 2
  line L165 (-40.0281, 35.9614) -> (-37.9532, 35.3921)
  spline S171 degree 2 poles (-37.9532, 35.3921) (-37.7766, 35.5916) (-37.5853, 35.9214) (-37.5274, 36.1324) knots 0 0 0 1 2 2 2
  spline S172 degree 2 poles (-37.5274, 36.1324) (-37.3998, 36.5974) (-37.9144, 37.31) (-38.6294, 37.5062) knots 0 0 0 1 2 2 2
  line L166 (-35.5999, 41.0559) -> (-35.7841, 40.4512)
  line L167 (-35.7841, 40.4512) -> (-36.1794, 40.5717)
  spline S173 degree 2 poles (-36.1794, 40.5717) (-36.0203, 40.2182) (-35.9207, 39.6415) (-36.0152, 39.3314) knots 0 0 0 1 2 2 2
  spline S174 degree 2 poles (-36.0152, 39.3314) (-36.086, 39.0988) (-36.3675, 38.7313) (-36.5802, 38.631) knots 0 0 0 1 2 2 2
  spline S175 degree 2 poles (-36.5802, 38.631) (-36.7941, 38.5267) (-37.3538, 38.5109) (-37.7181, 38.6219) knots 0 0 0 1 2 2 2
  line L168 (-37.7181, 38.6219) -> (-40.0476, 39.3317)
  line L169 (-40.0476, 39.3317) -> (-39.8633, 39.9363)
  line L170 (-39.8633, 39.9363) -> (-37.8168, 39.3128)
  spline S176 degree 2 poles (-37.8168, 39.3128) (-37.53, 39.2254) (-37.1411, 39.1534) (-36.9791, 39.1846) knots 0 0 0 1 2 2 2
  spline S177 degree 2 poles (-36.9791, 39.1846) (-36.8171, 39.2157) (-36.6124, 39.4287) (-36.5404, 39.6651) knots 0 0 0 1 2 2 2
  spline S178 degree 2 poles (-36.5404, 39.6651) (-36.4731, 39.886) (-36.5727, 40.4628) (-36.6911, 40.7276) knots 0 0 0 1 2 2 2
  line L171 (-36.6911, 40.7276) -> (-39.3732, 41.5448)
  line L172 (-39.3732, 41.5448) -> (-39.189, 42.1495)
  line L173 (-39.189, 42.1495) -> (-35.5999, 41.0559)
  line L174 (-37.612, 44.7796) -> (-37.6221, 44.7488)
  spline S179 degree 2 poles (-37.6221, 44.7488) (-37.6642, 44.6859) (-37.7215, 44.5384) (-37.7558, 44.4345) knots 0 0 0 1 2 2 2
  spline S180 degree 2 poles (-37.7558, 44.4345) (-37.8358, 44.1921) (-37.7817, 43.6452) (-37.6451, 43.3611) knots 0 0 0 1 2 2 2
  line L175 (-37.6451, 43.3611) -> (-35.1172, 42.5265)
  line L176 (-35.1172, 42.5265) -> (-35.3154, 41.9262)
  line L177 (-35.3154, 41.9262) -> (-38.8782, 43.1026)
  line L178 (-38.8782, 43.1026) -> (-38.6801, 43.7028)
  line L179 (-38.6801, 43.7028) -> (-38.1491, 43.5275)
  spline S181 degree 2 poles (-38.1491, 43.5275) (-38.3335, 43.9511) (-38.4108, 44.5185) (-38.3345, 44.7494) knots 0 0 0 1 2 2 2
  spline S182 degree 2 poles (-38.3345, 44.7494) (-38.304, 44.8417) (-38.2659, 44.9315) (-38.2353, 44.9854) knots 0 0 0 1 2 2 2
  line L180 (-38.2353, 44.9854) -> (-37.612, 44.7796)
  spline S183 degree 2 poles (-33.9254, 44.2049) (-33.8769, 44.2564) (-33.7101, 44.4594) (-33.6227, 44.5961) knots 0 0 0 1 2 2 2
  spline S184 degree 2 poles (-33.6227, 44.5961) (-33.5223, 44.7453) (-33.3735, 45.0063) (-33.3151, 45.1704) knots 0 0 0 1 2 2 2
  spline S185 degree 2 poles (-33.3151, 45.1704) (-33.2173, 45.4452) (-33.2265, 45.8786) (-33.3182, 46.0317) knots 0 0 0 1 2 2 2
  spline S186 degree 2 poles (-33.3182, 46.0317) (-33.4113, 46.1809) (-33.7225, 46.382) (-33.9401, 46.4595) knots 0 0 0 1 2 2 2
  line L181 (-33.9401, 46.4595) -> (-34.2493, 46.5695)
  spline S187 degree 2 poles (-34.2493, 46.5695) (-34.1249, 46.2543) (-34.0908, 45.7217) (-34.2145, 45.3744) knots 0 0 0 1 2 2 2
  spline S188 degree 2 poles (-34.2145, 45.3744) (-34.4291, 44.7712) (-35.5803, 44.3767) (-36.4239, 44.6769) knots 0 0 0 1 2 2 2
  spline S189 degree 2 poles (-36.4239, 44.6769) (-36.8629, 44.8332) (-37.454, 45.3231) (-37.6212, 45.6149) knots 0 0 0 1 2 2 2
  spline S190 degree 2 poles (-37.6212, 45.6149) (-37.7757, 45.8935) (-37.8296, 46.5277) (-37.7263, 46.8178) knots 0 0 0 1 2 2 2
  spline S191 degree 2 poles (-37.7263, 46.8178) (-37.6285, 47.0927) (-37.3561, 47.4473) (-37.1657, 47.6075) knots 0 0 0 1 2 2 2
  line L182 (-37.1657, 47.6075) -> (-37.3024, 47.6948)
  line L183 (-37.3024, 47.6948) -> (-37.1027, 48.256)
  line L184 (-37.1027, 48.256) -> (-33.9725, 47.1419)
  spline S192 degree 2 poles (-33.9725, 47.1419) (-33.0716, 46.8213) (-32.5103, 45.7398) (-32.797, 44.9344) knots 0 0 0 1 2 2 2
  spline S193 degree 2 poles (-32.797, 44.9344) (-32.8893, 44.6748) (-33.1662, 44.1626) (-33.3178, 43.9542) knots 0 0 0 1 2 2 2
  line L185 (-33.3178, 43.9542) -> (-33.9362, 44.1743)
  line L186 (-33.9362, 44.1743) -> (-33.9254, 44.2049)
  line L187 (-34.7379, 46.7434) -> (-36.6809, 47.4349)
  spline S194 degree 2 poles (-36.6809, 47.4349) (-36.8666, 47.2516) (-37.0914, 46.9101) (-37.1579, 46.723) knots 0 0 0 1 2 2 2
  spline S195 degree 2 poles (-37.1579, 46.723) (-37.3183, 46.2726) (-36.8388, 45.517) (-36.2166, 45.2956) knots 0 0 0 1 2 2 2
  spline S196 degree 2 poles (-36.2166, 45.2956) (-35.6287, 45.0864) (-34.8742, 45.2608) (-34.7166, 45.7036) knots 0 0 0 1 2 2 2
  spline S197 degree 2 poles (-34.7166, 45.7036) (-34.6337, 45.9365) (-34.6431, 46.4903) (-34.7379, 46.7434) knots 0 0 0 1 2 2 2
  point P0 (0, 0)
  constraints: 2 point on circle, 1 centre point, 1 other
extrude "Extrusion3" add sketch "Skizze3" along normal blind 1
